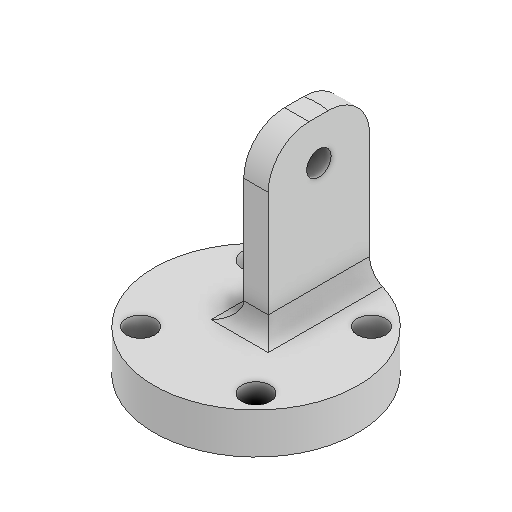
# Autodesk Inventor part: Base
Saved by Autodesk Inventor 2025.2 (Build 292293000, 293)
## iProperties
Created: 2025-05-03
Part Number: Base
Material: Genérico
Document SubType Name: Modeling
Designer: acer
Density: 1 g/cm^3
Appearance: Valor por defecto
Author: acer
Autodesk Inventor part; units mm, degrees
ref_plane "YZ Plane" through (0, 0, 0) normal (1, 0, 0) x (0, 1, 0)
ref_plane "XZ Plane" through (0, 0, 0) normal (0, 1, 0) x (-1, 0, 0)
ref_plane "XY Plane" through (0, 0, 0) normal (0, 0, 1) x (1, 0, 0)
sketch "Boceto1" plane through (0, 0, 0) normal (0, 1, 0) x (-1, 0, 0)
  circle A0 centre (14.1421, -14.1421) radius 3.5
  circle A1 centre (-14.1421, -14.1421) radius 3.5
  circle A2 centre (-14.1421, 14.1421) radius 3.5
  circle A3 centre (14.1421, 14.1421) radius 3.5
  circle A4 centre (0, 0) radius 25
  circle A5 centre (0, 0) radius 20
  dimension "d24" = 40
  dimension "d23" = 7
  dimension "d25" = 50
  dimension "d26" = 7
  dimension "d27" = 7
  dimension "d28" = 7
  constraints: 5 centre point, 1 coincident, 3 other
  measures "d23" diameter of A0
  measures "d25" diameter of A4
  measures "d26" diameter of A1
  measures "d27" diameter of A3
  measures "d28" diameter of A2
extrude "Extrusión1" add sketch "Boceto1" along normal blind 10 contours A0 A5 A1 A2 A3 | A4
sketch "Boceto2" plane through (0, 10, 0) normal (0, 1, 0) x (1, 0, 0)
  line L0 (0, 0) -> (3, 0)
  line L1 (3, 0) -> (3, 24.8193)
  circle A0 centre (0, 0) radius 25 projected
  line L2 (0, 0) -> (-3, 0)
  line L3 (-3, 0) -> (-3, 24.8193)
  arc A1 (3, 24.8193) -> (-3, 24.8193) centre (0, 0) ccw
  dimension "d13" = 3
  dimension "d14" = 3
  constraints: 8 end point, 4 point on circle, 2 perpendicular, 1 centre point, 1 coincident, 1 concentric, 1 horizontal, 1 point on line
  measures "d13" distance of L0.start L0.end
  measures "d14" distance of L2.start L2.end
extrude "Extrusión2" add sketch "Boceto2" along normal blind 40 contours L2 L3 A0 L1 L0 picked at (-2, 8.2731)
fillet "Empalme1" radius 10 1 edges at (0, 50, 0)
fillet "Empalme2" radius 10 1 edges at (0, 50, -25)
fillet "Empalme3" radius 4 3 edges at (3, 10, -12.4097) (0, 10, 0) (-3, 10, -12.4097)
sketch "Boceto3" plane through (3, 50, -10) normal (1, 0, 0) x (0, 0, -1)
  line L0 (-10, -36) -> (-10, -10) projected
  line L1 (14.8193, -36) -> (14.8193, -10) projected
  circle A0 centre (2.4097, -10) radius 3
  point P0 (-10, -50)
  constraints: 1 centre point
extrude "Extrusión3" cut sketch "Boceto3" against normal blind 40
